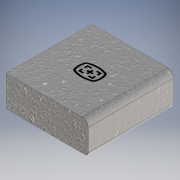
# Autodesk Inventor part: PRZYCISK IO
Saved by Autodesk Inventor 2017 SP1 (Build 210196100, 196)
## iProperties
Created: 2021-03-07
Part Number: PRZYCISK IO
Material: Tworzywo sztuczne, nieprzezroczyste czarne
Document SubType Name: Modeling
Designer: Administrator
Density: 0.952 g/cm^3
Appearance: Teksturowany - szary
Author: Administrator
Autodesk Inventor part; units mm, degrees
ref_plane "YZ Plane" through (0, 0, 0) normal (1, 0, 0) x (0, 1, 0)
ref_plane "XZ Plane" through (0, 0, 0) normal (0, 1, 0) x (-1, 0, 0)
ref_plane "XY Plane" through (0, 0, 0) normal (0, 0, 1) x (1, 0, 0)
sketch "Szkic1" plane through (0, 0, 0) normal (0, 0, 1) x (1, 0, 0)
  line L0 (206.45, -143.65) -> (206.45, -129.275)
  line L1 (206.45, -129.275) -> (220.2, -129.275)
  line L2 (206.45, -143.65) -> (220.2, -143.65)
  line L3 (220.2, -129.275) -> (220.2, -143.65)
  constraints: 8 end point
extrude "Wyciągnięcie proste1" add sketch "Szkic1" against normal blind 5.2
fillet "Zaokrąglenie1" radius 0.5 1 edges at (220.2, -136.4625, -5.2)
sketch "Szkic6" plane through (0, 0, 0) normal (0, 0, 1) x (1, 0, 0)
  line L0 (213.825, -136.3125) -> (213.825, -136.6125)
  line L1 (212.825, -136.6125) -> (212.825, -136.3125)
  line L2 (213.175, -135.9625) -> (213.475, -135.9625)
  line L3 (213.475, -136.9625) -> (213.175, -136.9625)
  line L4 (213.825, -136.6125) -> (213.475, -136.6125)
  line L5 (213.175, -136.6125) -> (212.825, -136.6125)
  line L6 (213.175, -136.9625) -> (213.175, -136.6125)
  line L7 (213.175, -136.3125) -> (213.175, -135.9625)
  line L8 (213.475, -135.9625) -> (213.475, -136.3125)
  line L9 (213.475, -136.6125) -> (213.475, -136.9625)
  line L10 (212.825, -136.3125) -> (213.175, -136.3125)
  line L11 (213.475, -136.3125) -> (213.825, -136.3125)
  line L12 (212.9, -137.2903) -> (212.1, -137.2903)
  line L13 (212.1, -137.2903) -> (212.1, -136.6403)
  line L14 (212.1, -136.6403) -> (212.4, -136.6403)
  line L15 (212.4, -136.6403) -> (212.4, -137.0153)
  line L16 (212.4, -137.0153) -> (212.9, -137.0153)
  line L17 (212.9, -137.0153) -> (212.9, -137.2903)
  line L18 (213.75, -137.2903) -> (214.55, -137.2903)
  line L19 (214.55, -137.2903) -> (214.55, -136.6403)
  line L20 (214.55, -136.6403) -> (214.25, -136.6403)
  line L21 (214.25, -136.6403) -> (214.25, -137.0153)
  line L22 (214.25, -137.0153) -> (213.75, -137.0153)
  line L23 (213.75, -137.0153) -> (213.75, -137.2903)
  line L24 (212.9, -135.6347) -> (212.1, -135.6347)
  line L25 (212.1, -135.6347) -> (212.1, -136.2847)
  line L26 (212.1, -136.2847) -> (212.4, -136.2847)
  line L27 (212.4, -136.2847) -> (212.4, -135.9097)
  line L28 (212.4, -135.9097) -> (212.9, -135.9097)
  line L29 (212.9, -135.9097) -> (212.9, -135.6347)
  line L30 (213.75, -135.9097) -> (213.75, -135.6347)
  line L31 (214.25, -136.2847) -> (214.25, -135.9097)
  line L32 (214.25, -135.9097) -> (213.75, -135.9097)
  line L33 (214.55, -136.2847) -> (214.25, -136.2847)
  line L34 (214.55, -135.6347) -> (214.55, -136.2847)
  line L35 (213.75, -135.6347) -> (214.55, -135.6347)
  arc A0 (211.7792, -135.6557) -> (211.7792, -137.2693) centre (213.8094, -136.4625) ccw
  arc A1 (214.7263, -135.514) -> (211.9237, -135.514) centre (213.325, -139.2478) ccw
  arc A2 (211.9237, -137.411) -> (214.7263, -137.411) centre (213.325, -133.6772) ccw
  arc A3 (214.8708, -137.2693) -> (214.8708, -135.6557) centre (212.8406, -136.4625) ccw
  arc A4 (215.1708, -137.2693) -> (215.1708, -135.6557) centre (213.1406, -136.4625) ccw
  arc A5 (215.1776, -135.6727) -> (214.7263, -135.214) centre (214.4204, -135.9663) ccw
  arc A6 (214.7263, -137.711) -> (215.1776, -137.2523) centre (214.4204, -136.9587) ccw
  arc A7 (211.9237, -135.514) -> (211.7792, -135.6557) centre (212.0023, -135.7386) ccw
  arc A8 (211.7792, -137.2693) -> (211.9237, -137.411) centre (212.0023, -137.1864) ccw
  arc A9 (214.8708, -135.6557) -> (214.7263, -135.514) centre (214.6477, -135.7386) ccw
  arc A10 (214.7263, -137.411) -> (214.8708, -137.2693) centre (214.6477, -137.1864) ccw
  arc A11 (211.4912, -135.5391) -> (211.4912, -137.3859) centre (213.9698, -136.4625) ccw
  arc A12 (213.325, -134.9597) -> (211.7797, -135.2472) centre (213.3235, -139.2481) ccw
  arc A13 (211.7797, -135.2472) -> (211.4912, -135.5391) centre (211.9597, -135.7137) ccw
  arc A14 (211.7797, -137.6778) -> (213.325, -137.9653) centre (213.3235, -133.6769) ccw
  arc A15 (211.4912, -137.3859) -> (211.7797, -137.6778) centre (211.9597, -137.2113) ccw
  arc A16 (215.1588, -137.3859) -> (215.1588, -135.5391) centre (212.6802, -136.4625) ccw
  arc A17 (214.8703, -135.2472) -> (213.325, -134.9597) centre (213.3265, -139.2481) ccw
  arc A18 (215.1588, -135.5391) -> (214.8703, -135.2472) centre (214.6903, -135.7137) ccw
  arc A19 (213.325, -137.9653) -> (214.8703, -137.6778) centre (213.3265, -133.6769) ccw
  arc A20 (214.8703, -137.6778) -> (215.1588, -137.3859) centre (214.6903, -137.2113) ccw
  point P0 (213.325, -136.4625)
  dimension "d56" = 0.3
  dimension "d63" = 0.65
  dimension "d64" = 0.3
  dimension "d66" = 0.375
  dimension "d68" = 0.5
  constraints: 72 end point, 42 point on circle, 21 centre point, 10 parallel, 6 perpendicular, 4 vertical, 3 horizontal, 2 tangent
  measures "d56" distance of L0.start L0.end
  measures "d63" distance of L12.end L13.end
  measures "d64" distance of L13.end L14.end
  measures "d66" distance of L14.end L15.end
  measures "d68" distance of L15.end L16.end
fillet "Zaokrąglenie2" radius 1 1 edges at (220.2, -136.4625, 0)
extrude "Wyciągnięcie proste5" add sketch "Szkic6" along normal blind 0.001
